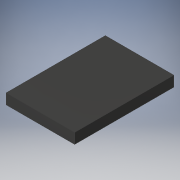
# Autodesk Inventor part: tampa caixa
Saved by Autodesk Inventor 2019.4 (Build 234330000, 330)
## iProperties
Created: 2021-02-25
Part Number: tampa caixa
Material: PCL plástico
Document SubType Name: Modeling
Designer: Lattes
Density: 1.626 g/cm^3
Appearance: Liso - Preto
Author: Lattes
Autodesk Inventor part; units mm, degrees
ref_plane "YZ Plane" through (0, 0, 0) normal (1, 0, 0) x (0, 1, 0)
ref_plane "XZ Plane" through (0, 0, 0) normal (0, 1, 0) x (-1, 0, 0)
ref_plane "XY Plane" through (0, 0, 0) normal (0, 0, 1) x (1, 0, 0)
sketch "Esboço1" plane through (0, 0, 0) normal (0, 1, 0) x (-1, 0, 0)
  line L0 (3, 3) -> (182, 3)
  line L1 (3, 262) -> (182, 262)
  line L2 (182, 262) -> (182, 3)
  line L3 (182, 3) -> (3, 3)
  line L4 (3, 3) -> (3, 262)
  line L5 (6, 6) -> (179, 6)
  line L6 (179, 259) -> (6, 259)
  line L7 (179, 6) -> (6, 6)
  line L8 (6, 6) -> (6, 259)
  line L9 (6, 259) -> (179, 259)
  line L10 (179, 259) -> (179, 6)
  point P0 (0, 0)
  point P1 (0, 0)
  constraints: 22 end point, 4 parallel, 2 horizontal, 2 perpendicular
extrude "Extrusão1" add sketch "Esboço1" along normal blind 25
sketch "Esboço2" plane through (0, 25, 0) normal (0, 1, 0) x (1, 0, 0)
  line L0 (-182, -3) -> (-3, -3) projected
  line L1 (-3, -262) -> (-3, -3) projected
  line L2 (-182, -3) -> (-3, -3)
  line L3 (-3, -3) -> (-3, -262)
  line L4 (-3, -262) -> (-182, -262)
  line L5 (-182, -262) -> (-182, -3)
  point P0 (0, 0)
  constraints: 8 end point, 2 parallel, 1 horizontal, 1 perpendicular
extrude "Extrusão2" add sketch "Esboço2" along normal blind 2
